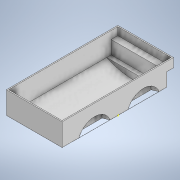
# Autodesk Inventor part: Karosserie
Saved by Autodesk Inventor 2021 (Build 250183000, 183)
## iProperties
Created: 2021-01-08
Part Number: Karosserie
Material: Generisch
Document SubType Name: Modeling
Designer: Jaro Machnow
Density: 1 g/cm^3
Appearance: Vorgabe
Author: Jaro Machnow
Autodesk Inventor part; units mm, degrees
ref_plane "YZ Plane" through (0, 0, 0) normal (1, 0, 0) x (0, 1, 0)
sketch "Skizze1" plane through (0, 0, 0) normal (0, 1, 0) x (-1, 0, 0)
  line L0 (1250, 2500) -> (-1250, 2500)
  line L1 (-1250, 2500) -> (-1250, -2500)
  line L2 (-1250, -2500) -> (1250, -2500)
  line L3 (1250, -2500) -> (1250, 2500)
  line L4 (1250, 0) -> (-1250, 0) construction
  line L5 (0, 2500) -> (0, -2500) construction
  point P0 (0, 0)
  dimension "Karosserie_Breite" = 2500
  dimension "Karosserie_Länge" = 5000
  constraints: 12 end point, 6 midpoint, 2 parallel, 1 horizontal, 1 perpendicular
  measures "Karosserie_Breite" distance of L2.end L1.end
  measures "Karosserie_Länge" distance of L1.end L0.end
extrude "Mitte" add sketch "Skizze1" along normal blind 1000
sketch "Skizze2" plane through (1250, 0, 2500) normal (1, 0, 0) x (0, 0, -1)
  line L0 (5000, 0) -> (5000, 1000) projected
  line L1 (5000, 0) -> (4700, 0)
  line L2 (4700, 0) -> (4700, 600)
  line L3 (4700, 600) -> (5000, 600)
  line L4 (5000, 600) -> (5000, 0)
  point P0 (2500, 0)
  dimension "Karosserie_Hinten_Minus_Tiefe" = 300
  dimension "Karosserie_Hinten_Minus_Höhe" = 600
  constraints: 8 end point, 2 parallel, 1 horizontal, 1 perpendicular
  measures "Karosserie_Hinten_Minus_Tiefe" distance of L2.end L3.end
  measures "Karosserie_Hinten_Minus_Höhe" distance of L1.end L2.end
extrude "Hinten_Minus" cut sketch "Skizze2" against normal through all
sketch "Skizze3" plane through (0, 0, 0) normal (0, 0, 1) x (1, 0, 0)
  arc A0 (-1250, 0) -> (1253.833, 0) centre (1.9165, 2726.2988) ccw
  line L0 (-1250, 0) -> (-1250, 1000) projected
  line L1 (-1250, 0) -> (1253.833, 0)
  point P0 (0, 0)
  dimension "Karosserie_Unten_Wölbung_Durchmesser" = 3000
  constraints: 2 end point, 2 point on circle, 1 centre point, 1 perpendicular
  measures "Karosserie_Unten_Wölbung_Durchmesser" radius of A0
extrude "Unten_Wölbung" add sketch "Skizze3" along normal mid plane 4000
sketch "Skizze4" plane through (0, 1000, 0) normal (0, 1, 0) x (1, 0, 0)
  line L0 (-1250, 2500) -> (-1250, -2500) projected
  line L1 (1250, -2500) -> (1250, 2500) projected
  line L2 (-1250, -1038.0425) -> (1250, -1038.0425)
  line L3 (1250, -1038.0425) -> (1250, 1961.9575)
  line L4 (1250, 1961.9575) -> (-1250, 1961.9575)
  line L5 (-1250, 1961.9575) -> (-1250, -1038.0425)
  point P0 (0, 0)
  dimension "Karosserie_Oben_Länge" = 3000
  constraints: 8 end point, 2 parallel, 2 point on line, 1 horizontal, 1 perpendicular
  measures "Karosserie_Oben_Länge" distance between parallel lines of L4 L2
ref_plane "Arbeitsebene2" through (1250, 1800, 2500) normal (0, 1, 0) x (1, 0, 0)
ref_plane "Arbeitsebene1" through (1250, 1000, 2500) normal (0, 1, 0) x (1, 0, 0)
sketch "Skizze5" plane through (1250, 1800, 2500) normal (0, 1, 0) x (1, 0, 0)
  line L0 (-2500, 5000) -> (-2500, 0) projected
  line L1 (0, 0) -> (0, 5000) projected
  line L2 (-2150, 2178.934) -> (-350, 2178.934)
  line L3 (-350, 2178.934) -> (-350, 4178.934)
  line L4 (-350, 4178.934) -> (-2150, 4178.934)
  line L5 (-2150, 4178.934) -> (-2150, 2178.934)
  line L6 (-1250, 2178.934) -> (-1250, 4178.934) construction
  point P0 (-1250, 2500)
  dimension "Karosserie_Oben_Dach_Länge" = 2000
  dimension "Karosserie_Oben_Dach_Breite" = 1800
  constraints: 10 end point, 2 midpoint, 2 parallel, 1 horizontal, 1 perpendicular, 1 point on line
  measures "Karosserie_Oben_Dach_Länge" distance of L4.end L2.start
  measures "Karosserie_Oben_Dach_Breite" distance of L3.end L4.end
feature "Oben" [suppressed]
sketch "Skizze6" plane through (1250, 0, 2500) normal (1, 0, 0) x (0, 0, -1)
  point P0 (2500, 0)
ref_plane "Arbeitsebene3" through (1250, 1000, 2500) normal (1, 0, 0) x (0, 0, -1)
sketch "Skizze7" plane through (1250, 1000, 2500) normal (1, 0, 0) x (0, 0, -1)
  line L0 (4500, -1273.7012) -> (500, -1273.7012) projected
  line L1 (500, -1000) -> (500, -1273.7012) projected
  line L2 (4500, -1273.7012) -> (4500, -1000) projected
  line L3 (500, -1000) -> (4500, -1000) projected
  arc A0 (2206.3143, -1273.7012) -> (706.3143, -1273.7012) centre (1456.3143, -1273.7012) ccw
  line L4 (706.3143, -1273.7012) -> (2206.3143, -1273.7012)
  arc A1 (4406.3143, -1273.7012) -> (2906.3143, -1273.7012) centre (3656.3143, -1273.7012) ccw
  line L5 (2906.3143, -1273.7012) -> (4406.3143, -1273.7012)
  point P0 (2500, -1000)
  dimension "Karosserie_Radaussparung_Breite" = 1600
  dimension "Karosserie_Radaussparung_Höhe" = 750
  dimension "d21" = 1600
  dimension "d22" = 750
  dimension "Karosserie_Radaussparung_Abstand" = 700
  constraints: 4 end point, 4 point on circle, 2 centre point, 2 point on line, 1 collinear
  measures "Karosserie_Radaussparung_Höhe" radius of A0
  measures "d22" radius of A1
  measures "Karosserie_Radaussparung_Abstand" distance of L5.start L4.end
extrude "Extrusion4" cut sketch "Skizze7" against normal blind 400 contours L0 A1 L3 | L3 A1 | L0 A0 L3 | L3 A0
sketch "Skizze8" plane through (1250, 1000, 2500) normal (0, 1, 0) x (1, 0, 0)
  line L0 (-2450, 50) -> (-50, 50)
  line L1 (-50, 50) -> (-50, 4950)
  line L2 (-50, 4950) -> (-2450, 4950)
  line L3 (-2450, 4950) -> (-2450, 50)
  line L4 (-2500, 5000) -> (-2500, 0) projected
  line L5 (-2500, 0) -> (0, 0) projected
  line L6 (0, 0) -> (0, 5000) projected
  line L7 (0, 5000) -> (-2500, 5000) projected
  line L8 (-2500, 0) -> (0, 0) construction
  line L9 (-1250, 0) -> (-1250, 5000) construction
  line L10 (-2500, 4500) -> (-2500, 500) construction
  line L11 (-2500, 2500) -> (0, 2500) construction
  line L12 (0, 2154.589) -> (0, 2958.0395) construction
  point P0 (-1250, 2500)
  dimension "Innen" = 50
  dimension "d27" = 50
  constraints: 12 end point, 3 midpoint, 2 parallel, 2 perpendicular, 1 horizontal, 1 point on line, 2 other
  measures "Innen" distance between parallel lines of L3 L4
  measures "d27" distance between parallel lines of L7 L2
shell "Wandung1" thickness 1 removed faces 0
extrude "Extrusion5" cut sketch "Skizze8" against normal blind 200 contours L3 L2 L1 L0
equation "\"d21\" = Karosserie_Radaussparung_Breite"
equation "\"d22\" = Karosserie_Radaussparung_Höhe"
equation "\"d27\" = Innen"
